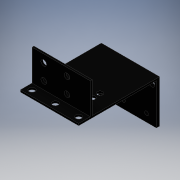
# Autodesk Inventor part: TrolleyLeftPlate1
Saved by Autodesk Inventor 2016 (Build 200138000, 138)
## iProperties
Created: 2016-03-28
Part Number: TrolleyLeftPlate1
Material: UHMW, Black
Document SubType Name: Modeling
Designer: mkepler
Density: 0.94 g/cm^3
Appearance: Smooth - Black
Mass: 8.44805 g
Surface Area: 111.05 cm^2
Volume: 8.98728 cm^3
Author: mkepler
Autodesk Inventor part; units mm, degrees
ref_plane "YZ Plane" through (0, 0, 0) normal (1, 0, 0) x (0, 1, 0)
ref_plane "XZ Plane" through (0, 0, 0) normal (0, 1, 0) x (-1, 0, 0)
ref_plane "XY Plane" through (0, 0, 0) normal (0, 0, 1) x (1, 0, 0)
sketch "Sketch1" plane through (0, 0, 0) normal (0, 1, 0) x (-1, 0, 0)
  line L0 (0, 0) -> (45, 0)
  line L1 (45, 0) -> (45, 31.5)
  line L2 (45, 31.5) -> (0, 31.5)
  line L3 (0, 31.5) -> (0, 0)
  dimension "d0" = 45
  dimension "d1" = 31.5
  constraints: 8 end point, 2 parallel, 1 horizontal, 1 perpendicular
  measures "d0" distance of L2.end L1.end
  measures "d1" distance of L1.end L0.end
extrude "Extrusion1" add sketch "Sketch1" along normal blind 2.5
sketch "Sketch2" plane through (0, 0, 0) normal (0, -1, 0) x (1, 0, 0)
  line L0 (-45, 0) -> (-45, 31.5) projected
  line L1 (-45, 31.5) -> (0, 31.5)
  line L2 (0, 31.5) -> (0, 33)
  line L3 (0, 33) -> (-45, 33)
  line L4 (-45, 33) -> (-45, 31.5)
  point P0 (0, 0)
  dimension "d4" = 45
  dimension "d5" = 1.5
  constraints: 8 end point, 2 parallel, 1 horizontal, 1 perpendicular
  measures "d4" distance of L3.end L2.end
  measures "d5" distance of L2.end L1.end
extrude "Extrusion2" add sketch "Sketch2" along normal blind 60 and the other way blind 2.5
sketch "Sketch4" plane through (0, 0, 0) normal (0, -1, 0) x (1, 0, 0)
  circle A0 centre (-3.5, 28) radius 2.3
  line L0 (-45, 31.5) -> (0, 31.5) projected
  line L1 (0, 31.5) -> (0, 0) projected
  line L2 (0, 0) -> (-45, 0) projected
  circle A1 centre (-41.5, 28) radius 2.3
  line L3 (-45, 0) -> (-45, 31.5) projected
  circle A2 centre (-41.5, 3.5) radius 2.3
  dimension "d10" = 4.6
  dimension "d11" = 3.5
  dimension "d12" = 3.5
  dimension "d16" = 4.6
  dimension "d17" = 3.5
  dimension "d18" = 3.5
  dimension "d19" = 4.6
  dimension "d20" = 3.5
  dimension "d21" = 3.5
  constraints: 3 centre point
  measures "d10" diameter of A0
  measures "d11" distance from line of L0 A0.centre
  measures "d12" distance from line of L1 A0.centre
  measures "d16" diameter of A1
  measures "d17" distance from line of L3 A1.centre
  measures "d18" distance from line of L0 A1.centre
  measures "d19" diameter of A2
  measures "d20" distance from line of A2.centre L2
  measures "d21" distance from line of L3 A2.centre
hole "Hole1" at (-3.5, 0, 28) at (-41.5, 0, 28) at (-41.5, 0, 3.5) direction (0, 1, 0) diameter 4.6 end through all
sketch "Sketch5" plane through (-45, -60, 33) normal (0, 0, 1) x (1, 0, 0)
  circle A0 centre (4.5, 4.5) radius 2.15
  line L0 (45, 0) -> (0, 0) projected
  line L1 (0, 62.5) -> (0, 0) projected
  circle A1 centre (40.5, 4.5) radius 2.15
  line L2 (45, 62.5) -> (45, 0) projected
  circle A2 centre (22.5, 4.5) radius 2.15
  point P0 (45, 60)
  dimension "d29" = 4.3
  dimension "d30" = 4.5
  dimension "d31" = 4.5
  dimension "d32" = 4.3
  dimension "d33" = 4.5
  dimension "d34" = 4.5
  dimension "d35" = 4.3
  constraints: 3 centre point
  measures "d29" diameter of A0
  measures "d30" distance from line of L0 A0.centre
  measures "d31" distance from line of L1 A0.centre
  measures "d32" diameter of A1
  measures "d33" distance from line of L2 A1.centre
  measures "d34" distance from line of L0 A1.centre
  measures "d35" diameter of A2
hole "Hole2" at (-40.5, -55.5, 33) at (-4.5, -55.5, 33) at (-22.5, -55.5, 33) direction (0, 0, -1) diameter 4.6 end through all
sketch "Sketch6" plane through (-45, -60, 33) normal (0, 0, 1) x (1, 0, 0)
  circle A0 centre (4.5, 4.5) radius 2.3 projected
  line L0 (4.5, 4.5) -> (4.5, 9)
  line L1 (0, 0) -> (0, 60) projected
  line L2 (0, 9) -> (45, 9)
  line L3 (45, 9) -> (45, 10.5)
  line L4 (45, 60) -> (45, 0) projected
  line L5 (45, 10.5) -> (0, 10.5)
  line L6 (0, 10.5) -> (0, 9)
  dimension "d43" = 4.5
  dimension "d44" = 1.5
  constraints: 10 end point, 3 point on line, 1 collinear, 1 horizontal, 1 perpendicular, 1 vertical
  measures "d43" distance of L0.start L0.end
  measures "d44" distance of L2.end L3.end
extrude "Extrusion3" add sketch "Sketch6" along normal blind 24 contours L1 L5 L3 L2
sketch "Sketch7" plane through (-45, 2.5, 33) normal (0, 0, 1) x (1, 0, 0)
  circle A0 centre (9, -40) radius 1.3
  line L0 (0, 0) -> (0, -52) projected
  line L1 (45, -52) -> (0, -52) projected
  circle A1 centre (33, -40) radius 2.15
  circle A2 centre (33, -34) radius 2.15
  circle A3 centre (33, -46) radius 2.15
  point P0 (45, -2.5)
  dimension "d47" = 2.6
  dimension "d48" = 9
  dimension "d49" = 12
  dimension "d50" = 4.3
  dimension "d51" = 24
  dimension "d52" = 4.3
  dimension "d53" = 6
  dimension "d54" = 4.3
  dimension "d55" = 6
  constraints: 4 centre point
  measures "d47" diameter of A0
  measures "d48" distance from line of L0 A0.centre
  measures "d49" distance from line of A0.centre L1
  measures "d50" diameter of A1
  measures "d51" distance of A1.centre A0.centre
  measures "d52" diameter of A2
  measures "d53" distance of A1.centre A2.centre
  measures "d54" diameter of A3
  measures "d55" distance of A3.centre A1.centre
hole "Hole3" at (-12, -31.5, 33) at (-12, -37.5, 33) at (-12, -43.5, 33) direction (0, 0, -1) diameter 4.3 end through all
sketch "Sketch8" plane through (-45, 2.5, 33) normal (0, 0, 1) x (1, 0, 0)
  circle A0 centre (33, -40) radius 2.15 projected
  line L0 (0, 0) -> (0, -52) projected
  circle A1 centre (9, -40) radius 1.3
  point P0 (45, -2.5)
  dimension "d89" = 2.6
  dimension "d91" = 9
  constraints: 1 centre point, 1 coincident
  measures "d89" diameter of A1
  measures "d91" distance from line of A1.centre L0
hole "Hole4" at (-12, -37.5, 33) at (-36, -37.5, 33) direction (0, 0, -1) diameter 2.6 end through all
sketch "Sketch9" plane through (-45, -49.5, 33) normal (0, 1, 0) x (1, 0, 0)
  circle A0 centre (9, -6) radius 2.15
  line L0 (0, 0) -> (45, 0) projected
  line L1 (0, 0) -> (0, -24) projected
  circle A1 centre (9, -18) radius 2.15
  circle A2 centre (27, -18) radius 2.15
  circle A3 centre (27, -6) radius 2.15
  point P0 (45, 33)
  dimension "d73" = 4.3
  dimension "d74" = 6
  dimension "d75" = 9
  dimension "d76" = 4.3
  dimension "d77" = 12
  dimension "d78" = 4.3
  dimension "d79" = 18
  dimension "d80" = 4.3
  dimension "d104" = 18
  dimension "d105" = 9
  constraints: 4 centre point
  measures "d73" diameter of A0
  measures "d74" distance from line of A0.centre L0
  measures "d75" distance from line of A0.centre L1
  measures "d76" diameter of A1
  measures "d77" distance of A0.centre A1.centre
  measures "d78" diameter of A2
  measures "d79" distance of A2.centre A1.centre
  measures "d80" diameter of A3
  measures "d104" distance of A3.centre A0.centre
  measures "d105" distance from line of L1 A1.centre
hole "Hole5" at (-36, -49.5, 39) at (-36, -49.5, 51) at (-18, -49.5, 51) at (-18, -49.5, 39) direction (0, -1, 0) diameter 4.3 end through all
sketch "Sketch10" plane through (0, 2.5, 0) normal (0, 1, 0) x (1, 0, 0)
  circle A0 centre (-7.5, -6) radius 1.5
  line L0 (0, 0) -> (-45, 0) projected
  line L1 (0, -33) -> (0, 0) projected
  circle A1 centre (-25.5, -6) radius 1.5
  dimension "d92" = 3
  dimension "d93" = 6
  dimension "d94" = 7.5
  dimension "d95" = 3
  dimension "d96" = 18
  constraints: 2 centre point
  measures "d92" diameter of A0
  measures "d93" distance from line of L0 A0.centre
  measures "d94" distance from line of L1 A0.centre
  measures "d95" diameter of A1
  measures "d96" distance of A1.centre A0.centre
hole "Hole6" at (-25.5, 2.5, 6) at (-7.5, 2.5, 6) direction (0, -1, 0) diameter 3 end through all
body "Solid1"
